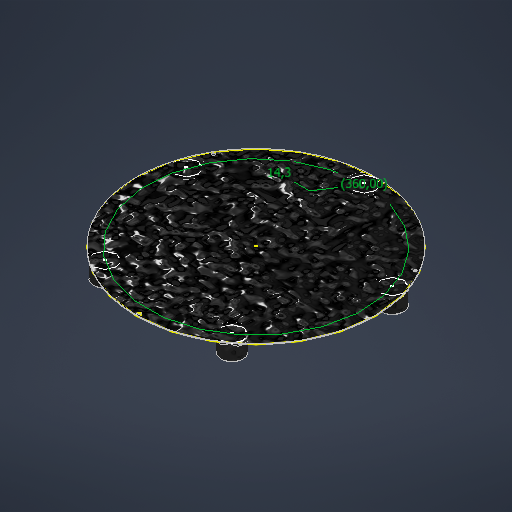
# Autodesk Inventor part: m2m_bottom_2
Saved by Autodesk Inventor 2026 (Build 300175000, 175)
## iProperties
Created: 2025-05-05
Part Number: m2m_bottom_2
Material: Generic
Document SubType Name: Modeling
Designer: Paul Juschitz
Density: 1 g/cm^3
Appearance: Black
Author: Paul Juschitz
Autodesk Inventor part; units mm, degrees
ref_plane "YZ Plane" through (0, 0, 0) normal (1, 0, 0) x (0, 1, 0)
ref_plane "XZ Plane" through (0, 0, 0) normal (0, 1, 0) x (-1, 0, 0)
ref_plane "XY Plane" through (0, 0, 0) normal (0, 0, 1) x (1, 0, 0)
derived "m2m_shell_3.ipt"
ref_plane "Work Plane1" through (0, 2, 0) normal (0, -1, 0) x (1, 0, 0)
sketch "Sketch3" plane through (0, 2, 0) normal (0, -1, 0) x (1, 0, 0)
  circle A0 centre (0, 0) radius 75.75
  dimension "d1" = 151.5
  constraints: 1 centre point, 1 coincident
  measures "d1" diameter of A0
extrude "Extrusion1" add sketch "Sketch3" along normal blind 0.5
sketch "Sketch4" plane through (0, 2, 0) normal (0, 1, 0) x (1, 0, 0)
  point P0 (0, 0)
  point P1 (0, -73.8904)
  point P2 (-63.991, 36.9452)
  point P3 (63.991, 36.9452)
hole "Hole1" at (-63.991, 2, -36.9452) at (63.991, 2, -36.9452) at (0, 2, 73.8904) direction (0, -1, 0) diameter 2 end through all
sketch "Sketch5" plane through (0, 1.5, 0) normal (0, -1, 0) x (1, 0, 0)
  circle A0 centre (0, -68.6) radius 7.15
  circle A1 centre (0, 73.8904) radius 1 projected
  circle A2 centre (0, 0) radius 75.75 projected
  circle A3 centre (65.2425, -21.1986) radius 7.15
  circle A4 centre (40.3221, 55.4986) radius 7.15
  circle A5 centre (-40.3221, 55.4986) radius 7.15
  circle A6 centre (-65.2425, -21.1986) radius 7.15
  dimension "m2m_bottom_foot_diameter" = 14.3
  dimension "d26" = 360
  constraints: 5 centre point, 1 tangent, 1 vertical alignment, 11 other
  measures "m2m_bottom_foot_diameter" diameter of A0
extrude "Extrusion2" add sketch "Sketch5" along normal blind 10.4 contours A0 | A3 | A4 | A5 | A6
fillet "Fillet1" radius 0.5 5 edges at (33.1721, -8.9, 55.4986) (58.0925, -8.9, -21.1986) (-7.15, -8.9, -68.6) (-72.3925, -8.9, -21.1986) (-47.4721, -8.9, 55.4986)
fillet "Fillet2" radius 2 10 edges at (-64.124, 1.5, -28.2605) (-66.361, 1.5, -14.1366) (5.0558, 1.5, -73.6558) (-5.0558, 1.5, -63.5442) (-43.5681, 1.5, 49.1279) (-37.076, 1.5, 61.8693) (72.3044, 1.5, -22.3171) (58.1805, 1.5, -20.0801) (33.9514, 1.5, 52.2525) (46.6928, 1.5, 58.7446)
sketch "Sketch2" plane through (0, 2, 0) normal (0, -1, 0) x (1, 0, 0)
  circle A0 centre (0, 73.8904) radius 1.25 projected
  circle A1 centre (0, 73.8904) radius 1.95 projected
  circle A2 centre (-63.991, -36.9452) radius 1.95 projected
  circle A3 centre (-63.991, -36.9452) radius 1.25 projected
  circle A4 centre (63.991, -36.9452) radius 1.95 projected
  circle A5 centre (63.991, -36.9452) radius 1.25 projected
  point P0 (0, 0)
  constraints: 1 other
equation "\"d7\" = -m2m_shell_bottom_screwhole_inset"
equation "\"m2m_shell_bottom_screwhole_inset\" = -2"
body "Solid1"
